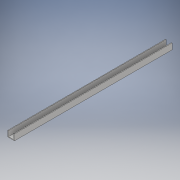
# Autodesk Inventor part: BackLiftProtoPart7
Saved by Autodesk Inventor 2017 (Build 210142000, 142)
## iProperties
Created: 2017-11-11
Part Number: BackLiftProtoPart7
Material: Generic
Document SubType Name: Modeling
Designer: User
Density: 1 g/cm^3
Appearance: Default
Author: User
Autodesk Inventor part; units mm, degrees
ref_plane "YZ Plane" through (0, 0, 0) normal (1, 0, 0) x (0, 1, 0)
ref_plane "XZ Plane" through (0, 0, 0) normal (0, 1, 0) x (-1, 0, 0)
ref_plane "XY Plane" through (0, 0, 0) normal (0, 0, 1) x (1, 0, 0)
sketch "Sketch1" plane through (0, 0, 0) normal (0, 0, 1) x (1, 0, 0)
  line L0 (0, 0) -> (0, -12.7)
  line L1 (0, -12.7) -> (12.7, -12.7)
  line L2 (12.7, -12.7) -> (12.7, 0)
  line L3 (12.7, 0) -> (14.2875, 0)
  line L4 (12.7, -14.2875) -> (14.2875, -14.2875)
  line L5 (14.2875, -14.2875) -> (14.2875, 0)
  line L6 (0, 0) -> (-1.5875, 0)
  line L7 (-1.5875, 0) -> (-1.5875, -14.2875)
  line L8 (-1.5875, -14.2875) -> (12.7, -14.2875)
  dimension "d0" = 12.7
  dimension "d2" = 1.5875
  dimension "d3" = 1.5875
  dimension "d4" = 1.5875
  constraints: 18 end point, 5 perpendicular, 1 horizontal, 1 parallel, 1 vertical
  measures "d0" distance of L0.start L0.end
  measures "d2" distance of L2.end L3.end
  measures "d3" distance of L1.end L4.start
  measures "d4" distance of L0.start L6.end
extrude "Extrusion1" add sketch "Sketch1" along normal blind 381
body "Solid1"
